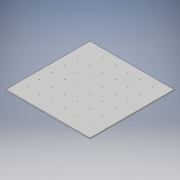
# Autodesk Inventor part: Bauteil1
Saved by Autodesk Inventor 2019 (Build 230136000, 136)
## iProperties
Created: 2021-09-26
Part Number: Bauteil1
Material: Generisch
Document SubType Name: Modeling
Designer: mritt
Density: 1 g/cm^3
Appearance: Vorgabe
Author: mritt
Autodesk Inventor part; units mm, degrees
ref_plane "YZ Plane" through (0, 0, 0) normal (1, 0, 0) x (0, 1, 0)
ref_plane "XZ Plane" through (0, 0, 0) normal (0, 1, 0) x (-1, 0, 0)
ref_plane "XY Plane" through (0, 0, 0) normal (0, 0, 1) x (1, 0, 0)
sketch "Skizze1" plane through (0, 0, 0) normal (0, 1, 0) x (-1, 0, 0)
  line L0 (2070.1754, -1385.0115) -> (70.1754, -1385.0115)
  line L1 (70.1754, -1385.0115) -> (70.1754, -3385.0115)
  line L2 (70.1754, -3385.0115) -> (2070.1754, -3385.0115)
  line L3 (2070.1754, -3385.0115) -> (2070.1754, -1385.0115)
  line L4 (370.1754, -1385.0115) -> (370.1754, -3385.0115)
  line L5 (670.1754, -3385.0115) -> (670.1754, -1385.0115)
  line L6 (970.1754, -1385.0115) -> (970.1754, -3385.0115)
  line L7 (1270.1754, -3385.0115) -> (1270.1754, -1385.0115)
  line L8 (1570.1754, -1385.0115) -> (1570.1754, -3385.0115)
  line L9 (70.1754, -1685.0115) -> (2070.1754, -1685.0115)
  line L10 (70.1754, -1985.0115) -> (2070.1754, -1985.0115)
  line L11 (70.1754, -2285.0115) -> (2070.1754, -2285.0115)
  line L12 (70.1754, -2585.0115) -> (2070.1754, -2585.0115)
  line L13 (70.1754, -2885.0115) -> (2070.1754, -2885.0115)
  line L14 (70.1754, -3185.0115) -> (2070.1754, -3185.0115)
  line L15 (1870.1754, -1385.0115) -> (1870.1754, -3385.0115)
  point P0 (0, 0)
  point P1 (1870.1754, -1685.0115)
  point P2 (1570.1754, -1685.0115)
  point P3 (1270.1754, -1685.0115)
  point P4 (970.1754, -1685.0115)
  point P5 (670.1754, -1685.0115)
  point P6 (370.1754, -1685.0115)
  point P7 (370.1754, -1985.0115)
  point P8 (670.1754, -1985.0115)
  point P9 (970.1754, -1985.0115)
  point P10 (1270.1754, -1985.0115)
  point P11 (1570.1754, -1985.0115)
  point P12 (1870.1754, -1985.0115)
  point P13 (1870.1754, -2285.0115)
  point P14 (1570.1754, -2285.0115)
  point P15 (1270.1754, -2285.0115)
  point P16 (970.1754, -2285.0115)
  point P17 (670.1754, -2285.0115)
  point P18 (370.1754, -2285.0115)
  point P19 (370.1754, -2585.0115)
  point P20 (670.1754, -2585.0115)
  point P21 (970.1754, -2585.0115)
  point P22 (1270.1754, -2585.0115)
  point P23 (1570.1754, -2585.0115)
  point P24 (1870.1754, -2585.0115)
  point P25 (1870.1754, -2885.0115)
  point P26 (1570.1754, -2885.0115)
  point P27 (1570.1754, -3185.0115)
  point P28 (1270.1754, -3185.0115)
  point P29 (1270.1754, -2885.0115)
  point P30 (970.1754, -2885.0115)
  point P31 (970.1754, -3185.0115)
  point P32 (670.1754, -3185.0115)
  point P33 (670.1754, -2885.0115)
  point P34 (370.1754, -2885.0115)
  point P35 (370.1754, -3185.0115)
  dimension "d0" = 2000
  dimension "d1" = 2000
  dimension "d2" = 300
  dimension "d3" = 300
  dimension "d4" = 300
  dimension "d5" = 300
  dimension "d6" = 300
  dimension "d8" = 300
  dimension "d9" = 300
  dimension "d10" = 300
  dimension "d11" = 300
  dimension "d12" = 300
  constraints: 84 point on line, 32 end point, 12 perpendicular, 2 parallel, 1 horizontal
  measures "d0" distance of L0.end L1.end
  measures "d1" distance of L1.end L2.end
  measures "d2" distance between parallel lines of L4 L1
  measures "d3" distance between parallel lines of L4 L5
  measures "d4" distance between parallel lines of L5 L6
  measures "d5" distance between parallel lines of L6 L7
  measures "d6" distance between parallel lines of L7 L8
  measures "d8" distance between parallel lines of L9 L0
  measures "d9" distance between parallel lines of L10 L9
  measures "d10" distance between parallel lines of L10 L11
  measures "d11" distance between parallel lines of L12 L11
  measures "d12" distance between parallel lines of L13 L12
extrude "Extrusion1" add sketch "Skizze1" along normal blind 20
extrude "Extrusion2" add sketch "Skizze1" along normal blind 20 contours L7 L11 L6 L10 | L6 L11 L5 L10 | L7 L12 L6 L11 | L6 L12 L5 L11
hole "Bohrung2" at (-1870.1754, 0, -1685.0115) at (-1570.1754, 0, -1685.0115) at (-1270.1754, 0, -1685.0115) at (-970.1754, 0, -1685.0115) at (-670.1754, 0, -1685.0115) at (-370.1754, 0, -1685.0115) at (-370.1754, 0, -1985.0115) at (-670.1754, 0, -1985.0115) at (-970.1754, 0, -1985.0115) at (-1270.1754, 0, -1985.0115) at (-1570.1754, 0, -1985.0115) at (-1870.1754, 0, -1985.0115) at (-1870.1754, 0, -2285.0115) at (-1570.1754, 0, -2285.0115) at (-1270.1754, 0, -2285.0115) at (-970.1754, 0, -2285.0115) at (-670.1754, 0, -2285.0115) at (-370.1754, 0, -2285.0115) at (-370.1754, 0, -2585.0115) at (-670.1754, 0, -2585.0115) at (-970.1754, 0, -2585.0115) at (-1270.1754, 0, -2585.0115) at (-1570.1754, 0, -2585.0115) at (-1870.1754, 0, -2585.0115) at (-1870.1754, 0, -2885.0115) at (-1570.1754, 0, -2885.0115) at (-1570.1754, 0, -3185.0115) at (-1270.1754, 0, -3185.0115) at (-1270.1754, 0, -2885.0115) at (-970.1754, 0, -2885.0115) at (-970.1754, 0, -3185.0115) at (-670.1754, 0, -3185.0115) at (-670.1754, 0, -2885.0115) at (-370.1754, 0, -3185.0115) at (-370.1754, 0, -2885.0115) direction (0, 1, 0) diameter 9.376 end through all thread size "M11x1.5" class "6H" standard "ANSI Metric M Profile"
